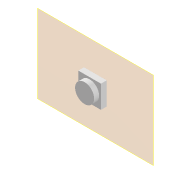
# Autodesk Inventor part: 00_ESP32_OmnivisionCameraModule
Saved by Autodesk Inventor 2022 (Build 260153000, 153)
## iProperties
Created: 2022-08-19
Part Number: 00_ESP32_OmnivisionCameraModule
Material: Generisch
Document SubType Name: Modeling
Designer: UC2
Density: 1 g/cm^3
Appearance: Vorgabe
Author: UC2
Autodesk Inventor part; units mm, degrees
ref_plane "YZ Plane" through (0, 0, 0) normal (1, 0, 0) x (0, 1, 0)
ref_plane "XZ Plane" through (0, 0, 0) normal (0, 1, 0) x (-1, 0, 0)
ref_plane "XY Plane" through (0, 0, 0) normal (0, 0, 1) x (1, 0, 0)
ref_plane "Arbeitsebene1" through (0, 0, 2.9972) normal (0, 0, 1) x (1, 0, 0)
sketch "Skizze1" plane through (0, 0, 2.9972) normal (0, 0, 1) x (1, 0, 0)
  circle A0 centre (-0.0001, 0.0021) radius 3 projected
  line L0 (4.2999, -4.2979) -> (-4.3001, -4.2979)
  line L1 (-4.3001, -4.2979) -> (-4.3001, 4.3021)
  line L2 (-4.3001, 4.3021) -> (4.2999, 4.3021)
  line L3 (4.2999, 4.3021) -> (4.2999, -4.2979)
  line L4 (4.2999, -4.2979) -> (-4.3001, 4.3021) construction
  line L5 (-4.3001, -4.2979) -> (4.2999, 4.3021) construction
  point P0 (0, 0)
  dimension "d0" = 8.6
  dimension "d1" = 8.6
  constraints: 12 end point, 2 midpoint, 2 parallel, 1 horizontal, 1 perpendicular
  measures "d0" distance of L1.end L2.end
  measures "d1" distance of L0.end L1.end
extrude "Extrusion1" add sketch "Skizze1" along normal blind 2.2 contours A0 | L0 L1 L2 L3
sketch "Skizze2" plane through (0, 0, 5.1972) normal (0, 0, 1) x (1, 0, 0)
  circle A0 centre (0, 0) radius 3.6
  dimension "d4" = 7.2
  constraints: 1 centre point, 1 coincident
  measures "d4" diameter of A0
extrude "Extrusion2" add sketch "Skizze2" along normal blind 1.9
